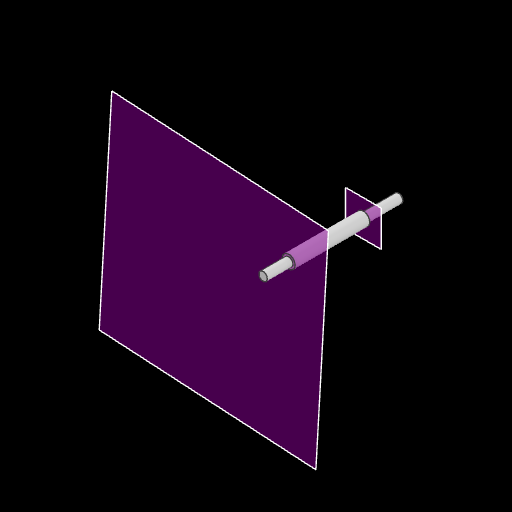
# Autodesk Inventor part: LegKneeShaft
Saved by Autodesk Inventor 2025.2 (Build 292293000, 293)
## iProperties
Created: 2025-11-09
Part Number: LegKneeShaft
Material: Generic
Document SubType Name: Modeling
Designer: valer
Density: 1 g/cm^3
Appearance: Default
Author: valer
Autodesk Inventor part; units mm, degrees
ref_plane "YZ Plane" through (0, 0, 0) normal (1, 0, 0) x (0, 1, 0)
ref_plane "XZ Plane" through (0, 0, 0) normal (0, 1, 0) x (-1, 0, 0)
ref_plane "XY Plane" through (0, 0, 0) normal (0, 0, 1) x (1, 0, 0)
sketch "Base" plane through (0, 0, 0) normal (0, 0, 1) x (1, 0, 0)
  line L0 (-3.5, 1.9365) -> (-3.5, -1.9365)
  line L1 (0, -5.6) -> (0, 5.6) construction
  circle A0 centre (0, 0) radius 4
  point P0 (-3.5, 0)
  dimension "d9" = 8
  dimension "d11" = 3.5
  constraints: 2 end point, 2 point on circle, 1 centre point, 1 coincident, 1 midpoint, 1 parallel
  measures "d9" diameter of A0
  measures "d11" distance from line of point (-3.5, 0) L1
ref_plane "BasePlane" through (-230.8476, -175.3438, -99) normal (0, 0, -1) x (0, 1, 0)
extrude "BaseFeature" add sketch "Base" against normal up to surface (99 mm away) contours A0 L0 picked at (-0.9569, 0.8781)
sketch "Sketch4" plane through (0, 0, 0) normal (0, 0, 1) x (1, 0, 0)
  line L0 (-3.5, 1.9365) -> (-3.5, -1.9365) projected
  arc A0 (-3.5, -1.9365) -> (-3.5, 1.9365) centre (0, 0) ccw projected
extrude "Extrusion4" add sketch "Sketch4" along normal blind 14
sketch "Sketch5" plane through (0, 0, -99) normal (0, 0, -1) x (-1, 0, 0)
  arc A0 (3.5, 1.9365) -> (3.5, -1.9365) centre (0, 0) ccw projected
  line L0 (3.5, 1.9365) -> (3.5, -1.9365) projected
  point P0 (0, 0)
extrude "Extrusion5" add sketch "Sketch5" along normal blind 14
ref_plane "Work Plane2" through (-70.1743, -50.75, -10) normal (0, 0, -1) x (-0.0587753, -0.9982712, 0)
ref_plane "Work Plane4" through (18.2792, 18.9137, -80) normal (0, 0, -1) x (0, 1, 0)
sketch "Sketch6" plane through (-70.1743, -50.75, -10) normal (0, 0, -1) x (-0.0587753, -0.9982712, 0)
  circle A0 centre (-54.7868, -67.0701) radius 4.165 projected
  circle A1 centre (-54.7868, -67.0701) radius 6
  point P0 (-54.7868, -67.0701)
  dimension "d16" = 12
  constraints: 1 centre point, 1 coincident
  measures "d16" diameter of A1
extrude "Extrusion6" add sketch "Sketch6" along normal up to surface (70 mm away) contours A0 | A1
body "Solid1"
